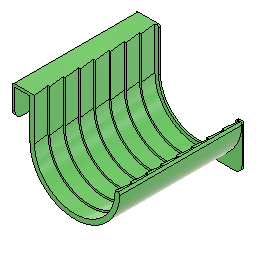
Lid Holder v8 (Autodesk Fusion 360 design; units mm, degrees)
Autodesk Fusion 360 part; units mm, degrees
note: some values were not read from the file. Set by a fixed rule: which sketch regions a step uses.
sketch "Sketch1" plane through (0, 0, 0) normal (0, 1, 0) x (1, 0, 0)
  line L0 (0, 0) -> (0, 30)
  line L1 (0, 30) -> (16, 30)
  line L2 (16, 30) -> (16, -12)
  line L3 (0, 0) -> (-3, 0)
  line L4 (-3, 0) -> (-3, 33)
  line L5 (-3, 33) -> (19, 33)
  line L6 (19, 33) -> (19, -12)
  line L7 (16, -12) -> (19, -12)
  line L8 (19, -12) -> (109, -12) construction
  arc A0 (19, -12) -> (109, -12) centre (64, -12) ccw
  arc A1 (16, -12) -> (112, -12) centre (64, -12) ccw
  line L9 (112, -12) -> (109, -12)
  dimension "d7" = 30
  dimension "d8" = 16
  dimension "d9" = 3
  dimension "d11" = 3
  dimension "d12" = 3
  dimension "d13" = 45
  dimension "d22" = 90
  constraint coincident L0.start L3.start
  constraint vertical L0
  constraint perpendicular L0 L1
  constraint perpendicular L1 L2
  constraint perpendicular L0 L3
  constraint perpendicular L3 L4
  constraint perpendicular L4 L5
  constraint perpendicular L5 L6
  constraint perpendicular L2 L7
  constraint perpendicular L6 L8
  constraint midpoint L8 A0.centre
  constraint coincident A0.centre A1.centre
  constraint parallel L8 L9
  measures "d7" distance of L0.start L0.end
  measures "d8" distance of L0.end L1.end
  measures "d9" distance of L0 L4
  measures "d11" distance of L2 L6
  measures "d12" distance of L1 L5
  measures "d13" distance of L5.end L6.end
  measures "d22" distance of L6.end L8.end
extrude "Extrude3" add sketch "Sketch1" along normal blind 130.4
sketch "Sketch4" plane through (0, 0, -33) normal (0, 0, -1) x (-1, 0, 0)
  line L0 (-19, 0) -> (3, 0)
  line L1 (3, 0) -> (3, 130.4)
  line L2 (3, 130.4) -> (-19, 130.4)
  line L3 (-19, 130.4) -> (-19, 0)
  line L4 (3, 0) -> (-19, 0)
  line L5 (3, 0) -> (3, 130.4)
  line L6 (-19, 130.4) -> (3, 130.4)
  line L7 (-19, 0) -> (-21, 0) construction
  line L8 (-21, 0) -> (-21, 130.4) construction
  line L9 (-19, 130.4) -> (-21, 130.4) construction
  line L10 (-19, 0) -> (-21, 16.3)
  line L11 (-19, 16.3) -> (-21, 16.3)
  line L12 (-19, 16.3) -> (-21, 32.6)
  line L13 (-19, 32.6) -> (-21, 32.6)
  line L14 (-19, 32.6) -> (-21, 48.9)
  line L15 (-19, 48.9) -> (-21, 48.9)
  line L16 (-16, 130.4) -> (-16, 0)
  line L17 (-19, 48.9) -> (-21, 65.2)
  line L18 (-19, 65.2) -> (-21, 65.2)
  line L19 (-19, 65.2) -> (-21, 81.5)
  line L20 (-19, 81.5) -> (-21, 81.5)
  line L21 (-19, 81.5) -> (-21, 97.8)
  line L22 (-19, 97.8) -> (-21, 97.8)
  line L23 (-19, 97.8) -> (-21, 114.1)
  line L24 (-19, 114.1) -> (-21, 114.1)
  line L25 (-19, 114.1) -> (-21, 130.4)
  line L26 (-19, 130.4) -> (-21, 130.4)
  dimension "d25" = 2
  dimension "d26" = 16.3
  dimension "d29" = 0
  dimension "d30" = 114.1
  constraint coincident L0.start L3.end
  constraint perpendicular L3 L7
  constraint perpendicular L7 L8
  constraint coincident L2.end L3.start
  constraint perpendicular L8 L9
  constraint coincident L8 L10.end
  constraint coincident L3 L11.start
  constraint perpendicular L8 L11
  constraint coincident L2 L16.start
  constraint coincident L4 L16.end
  constraint perpendicular L4 L16
  measures "d25" distance of L8.end L2.end
  measures "d26" distance of L0.start L11.start
sweep "Sweep1" add profiles "Sketch4" along 2 edges at (64, 130.4, 57) (19, 130.4, -10.5) section 1 contours L0 L2 L3 L4 L6 L16 | L3 L10 L11 | L3 L12 L13 | L3 L14 L15 | L3 L25 L26 | L3 L17 L18 | L3 L23 L24 | L3 L19 L20 | L3 L21 L22
sketch "Sketch5" plane through (0, 0, 0) normal (0, -1, 0) x (1, 0, 0)
  line L0 (16, -30) -> (0, -30)
  line L1 (0, -30) -> (0, 0)
  line L2 (0, 0) -> (-3, 0)
  line L3 (-3, 0) -> (-3, -33)
  line L4 (-3, -33) -> (19, -33)
  line L5 (19, -33) -> (19, 12)
  arc A0 (109, 12) -> (19, 12) centre (64, 12) ccw
  line L6 (109, 12) -> (112, 12)
  arc A1 (112, 12) -> (16, 12) centre (64, 12) ccw
  line L7 (16, 12) -> (16, -30)
  line L8 (23, -33) -> (23, 12)
  arc A2 (105, 12) -> (23, 12) centre (64, 12) ccw
  line L9 (23, -33) -> (19, -33)
  line L10 (105, 12) -> (109, 12)
  line L11 (16, 12) -> (16, 60)
  line L12 (16, 60) -> (112, 60)
  line L13 (112, 60) -> (112, 12)
  dimension "d40" = 4
  constraint coincident L4.end L5.start
  constraint perpendicular L5 L9
  constraint coincident A0.start L6.start
  constraint perpendicular L8 L10
  constraint coincident A1.end L7.start
  constraint tangent A1 L11
  constraint perpendicular L11 L12
  constraint coincident L6.end A1.start
  constraint perpendicular L6 L13
  constraint tangent A1 L12
extrude "Extrude4" add sketch "Sketch5" along normal blind 2
fillet "Fillet1" radius 8 2 edges at (112, -1, 60) (16, -1, 60)
fillet "Fillet2" radius 8 2 edges at (-1.5, -2, 0) (-1.5, 130.4, 0)
fillet "Fillet3" radius 2 3 edges at (-3, 64.2, -33) (112, 65.2, 12) (112, -1, 12)
fillet "Fillet3" radius 2 2 edges at (105, -1, 12) (23, -1, -33)
move_body "Move1" bodies 1 to x (1, 0, 0) y (0, 0, 1) z (0, -1, 0) at (-60, 60, -65)
equation "Overhang = 30 mm"
equation "DrawerWallThickness = 16 mm"
equation "LidDiameter = 90 mm"
equation "LidHeight = 16.3 mm"
equation "Clearance = 2 mm"
equation "SmallLidDiameter = 86 mm"
equation "d7 = Overhang"
equation "d8 = DrawerWallThickness"
equation "d9 = Thickness"
equation "Thickness = 3 mm"
equation "d11 = Thickness"
equation "d12 = Thickness"
equation "d13 = LidDiameter / 2"
equation "Count = 8"
equation "d22 = LidDiameter"
equation "d23 = LidHeight * Count"
equation "d25 = ( LidDiameter - SmallLidDiameter ) / 2"
equation "d26 = LidHeight"
equation "d28 = Count"
equation "d30 = LidHeight * ( Count - 1 )"
equation "d38 = EndLipThickness"
equation "d40 = EndLipHeight"
equation "EndLipHeight = 4 mm"
equation "EndLipThickness = 2 mm"
equation "LargeCornerRadius = 8 mm"
equation "d45 = LargeCornerRadius"
equation "d47 = LargeCornerRadius"
equation "SmallCornerRadius = 2 mm"
equation "d50 = SmallCornerRadius"
equation "d52 = SmallCornerRadius"
named bodies: "Lid Holder"
